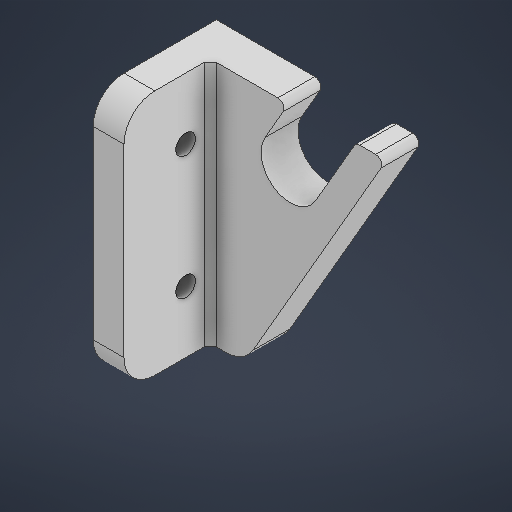
# Autodesk Inventor part: wheel holder
Saved by Autodesk Inventor 2026.1 (Build 301233020, 233B)
## iProperties
Created: 2025-12-29
Part Number: wheel holder
Material: Ogólny
Document SubType Name: Modeling
Designer: maciej
Density: 1 g/cm^3
Appearance: Domyślna
Author: maciej
Autodesk Inventor part; units mm, degrees
ref_plane "YZ Plane" through (0, 0, 0) normal (1, 0, 0) x (0, 1, 0)
ref_plane "XZ Plane" through (0, 0, 0) normal (0, 1, 0) x (-1, 0, 0)
ref_plane "XY Plane" through (0, 0, 0) normal (0, 0, 1) x (1, 0, 0)
sketch "Sketch1" plane through (0, 0, 0) normal (0, 0, 1) x (1, 0, 0)
  circle A0 centre (0, 0) radius 4.75
  circle A1 centre (0, 0) radius 9
  line L0 (-18, 9) -> (-18, -49.1769)
  line L1 (-18, 9) -> (10.681, 9)
  line L2 (4.1136, -2.375) -> (10.681, 9)
  line L3 (-0.2887, 9) -> (-4.1136, 2.375)
  line L4 (10.681, 9) -> (15.5885, 9)
  line L5 (4.1136, -2.375) -> (7.7942, -4.5) construction
  line L6 (7.7942, -4.5) -> (15.5885, 9)
  line L7 (7.7942, -4.5) -> (-18, -49.1769)
  line L8 (-18, -31) -> (-7.5056, -31)
  line L9 (-13, 9) -> (-13, -31)
  dimension "d1" = 18
  dimension "d0" = 9.5
  dimension "d2" = 18
  dimension "d5" = 120
  dimension "d7" = 60
  dimension "d8" = 40
  dimension "d9" = 5
  constraints: 20 end point, 5 point on line, 3 horizontal, 3 perpendicular, 2 coincident, 2 point on circle, 2 tangent, 1 centre point, 1 collinear, 1 parallel, 1 vertical, 3 other
  measures "d0" diameter of A0
  measures "d2" distance from line of L0 point (0, 0)
  measures "d5" angle of L1 L2
  measures "d7" angle of L1 L3
  measures "d8" distance between parallel lines of L1 L8
  measures "d9" distance between parallel lines of L0 L9
extrude "Extrusion1" add sketch "Sketch1" along normal blind 6 contours A0 L2 A1 L3 | A1 L7 L8 L9 L1 L3 | L2 L4 L6 A1 | L9 L8 L0 L1 picked at (-2.2884, 6.6758)
extrude "Extrusion2" add sketch "Sketch1" along normal blind 20 contours L9 L8 L0 L1
sketch "Sketch2" plane through (-18, -31, 0) normal (-1, 0, 0) x (0, 0, 1)
  line L0 (0, 40) -> (0, 0) projected
  line L1 (0, 0) -> (20, 0) projected
  line L2 (20, 40) -> (20, 0) projected
  line L3 (0, 40) -> (20, 40) projected
  circle A0 centre (10, 30) radius 1.6
  circle A1 centre (10, 10) radius 1.6
  point P0 (0, 31)
  dimension "d14" = 3.2
  dimension "d15" = 3.2
  dimension "d16" = 10
  dimension "d17" = 10
  dimension "d18" = 10
  constraints: 2 centre point, 1 vertical alignment
  measures "d14" diameter of A0
  measures "d15" diameter of A1
  measures "d16" distance from line of L2 A0.centre
  measures "d17" distance from line of L3 A0.centre
  measures "d18" distance from line of L1 A1.centre
extrude "Extrusion3" cut sketch "Sketch2" against normal blind 6 contours A0 | A1
fillet "Fillet1" radius 1 3 edges at (15.5885, 9, 3) (10.681, 9, 3) (-0.2887, 9, 3)
fillet "Fillet2" radius 5 3 edges at (-7.5056, -31, 3) (-15.5, -31, 20) (-15.5, 9, 20)
chamfer "Chamfer1" distance 1 angle 45 1 edges at (-13, -11, 6)
body "Solid1"
